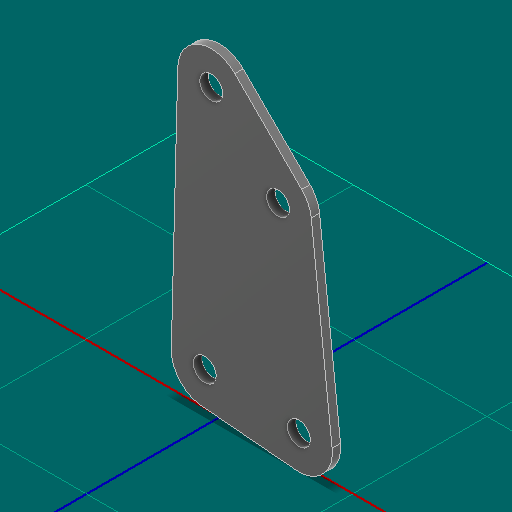
# Autodesk Inventor part: floating-stage-bracket
Saved by Autodesk Inventor 2025 (Build 290162000, 162)
## iProperties
Created: 2024-08-13
Part Number: floating-stage-bracket
Material: Acetal Resin, Black
Document SubType Name: Modeling
Designer: averey
Density: 1.425 g/cm^3
Appearance: Smooth - Black
Author: averey
Autodesk Inventor part; units mm, degrees
ref_plane "YZ Plane" through (0, 0, 0) normal (1, 0, 0) x (0, 1, 0)
ref_plane "XZ Plane" through (0, 0, 0) normal (0, 1, 0) x (-1, 0, 0)
ref_plane "XY Plane" through (0, 0, 0) normal (0, 0, 1) x (1, 0, 0)
sketch "main" plane through (0, 0, 0) normal (0, 0, 1) x (1, 0, 0)
  circle A0 centre (-9.3272, -22.4282) radius 2.1844
  circle A1 centre (8.5649, -23.9935) radius 2.1844
  circle A2 centre (4.5963, 11.9106) radius 2.1844
  arc A3 (-15.6751, -22.2631) -> (-9.3272, -28.7782) centre (-9.3272, -22.4282) ccw
  arc A4 (8.0027, -30.3186) -> (14.8765, -23.2959) centre (8.5649, -23.9935) ccw
  arc A5 (10.9079, 12.6083) -> (9.0865, 16.4007) centre (4.5963, 11.9106) ccw
  line L0 (-9.3272, -28.7782) -> (8.0027, -30.3186)
  line L1 (10.9079, 12.6083) -> (14.8765, -23.2959)
  circle A6 centre (-8.1037, 24.6106) radius 2.1844
  arc A7 (-3.6135, 29.1007) -> (-14.4515, 24.7757) centre (-8.1037, 24.6106) ccw
  line L2 (9.0865, 16.4007) -> (-3.6135, 29.1007)
  line L3 (-14.4515, 24.7757) -> (-15.6751, -22.2631)
  point P0 (-0.372, -2.6392)
  dimension "d0" = 12.7
  dimension "d1" = 12.7
  dimension "d2" = 12.7
  dimension "d3" = 12.7
  measures "d0" diameter of A3
  measures "d1" diameter of A4
  measures "d2" diameter of A5
  measures "d3" diameter of A7
sketch "Sketch1" plane through (0, 0, 0) normal (0, 0, 1) x (1, 0, 0)
  circle A0 centre (-1.2236, -47.0388) radius 2.1844
  circle A1 centre (16.6686, -48.6042) radius 2.1844
  circle A2 centre (12.7, -12.7) radius 2.1844
  arc A3 (-7.5714, -46.8737) -> (-1.2236, -53.3888) centre (-1.2236, -47.0388) ccw
  arc A4 (16.1064, -54.9292) -> (22.9802, -47.9065) centre (16.6686, -48.6042) ccw
  arc A5 (19.0116, -12.0024) -> (17.1901, -8.2099) centre (12.7, -12.7) ccw
  line L0 (-1.2236, -53.3888) -> (16.1064, -54.9292)
  line L1 (19.0116, -12.0024) -> (22.9802, -47.9065)
  circle A6 centre (0, 0) radius 2.1844
  arc A7 (4.4901, 4.4901) -> (-6.3479, 0.1651) centre (0, 0) ccw
  line L2 (17.1901, -8.2099) -> (4.4901, 4.4901)
  line L3 (-6.3479, 0.1651) -> (-7.5714, -46.8737)
  constraints: 1 other
extrude "Extrusion1" add sketch "Sketch1" along normal blind 1.5875
body "Solid1"
